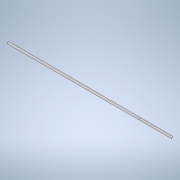
# Autodesk Inventor part: Part10
Saved by Autodesk Inventor 2022 (Build 260153000, 153)
## iProperties
Created: 2021-12-09
Part Number: Part10
Material: Generic
Document SubType Name: Modeling
Designer: keemi
Density: 1 g/cm^3
Appearance: Default
Author: keemi
Autodesk Inventor part; units mm, degrees
ref_plane "YZ Plane" through (0, 0, 0) normal (1, 0, 0) x (0, 1, 0)
ref_plane "XZ Plane" through (0, 0, 0) normal (0, 1, 0) x (-1, 0, 0)
ref_plane "XY Plane" through (0, 0, 0) normal (0, 0, 1) x (1, 0, 0)
sketch "Sketch1" plane through (0, 0, 0) normal (1, 0, 0) x (0, 1, 0)
  line L0 (0, 0) -> (50, 0) construction
  line L1 (50, 50) -> (0, 0)
  line L2 (50, 50) -> (52.1213, 47.8787)
  line L3 (0, 0) -> (2.1213, -2.1213)
  line L4 (2.1213, -2.1213) -> (52.1213, 47.8787)
  dimension "d4" = 3
  dimension "d5" = 3
  constraints: 10 end point, 2 perpendicular, 1 horizontal, 1 point on line
  measures "d4" distance of L1.start L2.end
  measures "d5" distance of L0.start L3.end
extrude "Extrusion1" add sketch "Sketch1" along normal blind 200
body "Solid1"
